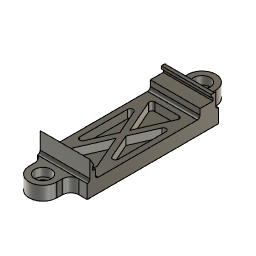
Relay support (Autodesk Fusion 360 design; units mm, degrees)
Autodesk Fusion 360 part; units mm, degrees
sketch "Sketch1" plane through (0, 0, 0) normal (1, 0, 0) x (0, 1, 0)
  line L0 (0, 0) -> (43.2, 0) construction
  line L1 (43.2, 0) -> (43.2, 1.2) construction
  line L2 (43.2, 1.2) -> (0, 1.2) construction
  line L3 (0, 1.2) -> (0, 0) construction
  line L4 (1.3, 0) -> (38.2, 0) construction
  line L5 (38.2, 0) -> (38.2, -2.6) construction
  line L6 (38.2, -2.6) -> (1.3, -2.6) construction
  line L7 (1.3, -2.6) -> (1.3, 0) construction
  line L8 (0.3, 1.4) -> (-1.2, 3.9981)
  line L9 (-1.2, 3.9981) -> (-1.2, -2.1)
  line L10 (-2.2, -3.1) -> (-12.2, -3.1)
  line L11 (-12.2, -3.1) -> (-12.2, -8.1)
  line L12 (-12.2, -8.1) -> (55.4, -8.1)
  line L13 (55.4, -8.1) -> (55.4, -3.1)
  line L14 (55.4, -3.1) -> (45.4, -3.1)
  line L15 (44.4, -2.1) -> (44.4, 1.9)
  line L16 (42.7, 1.4) -> (43.1, 1.4)
  line L17 (43.4, 1.1) -> (43.4, 0)
  line L18 (0.3, 1.4) -> (0.1, 1.4)
  line L19 (-0.2, 1.1) -> (-0.2, 0)
  line L20 (-0.2, 0) -> (0.8, 0)
  line L21 (0.8, 0) -> (0.8, -2.1)
  line L22 (1.8, -3.1) -> (37.7, -3.1)
  line L23 (38.7, -2.1) -> (38.7, 0)
  line L24 (38.7, 0) -> (43.4, 0)
  arc A0 (-2.2, -3.1) -> (-1.2, -2.1) centre (-2.2, -2.1) ccw
  arc A1 (44.4, -2.1) -> (45.4, -3.1) centre (45.4, -2.1) ccw
  arc A2 (0.8, -2.1) -> (1.8, -3.1) centre (1.8, -2.1) ccw
  arc A3 (37.7, -3.1) -> (38.7, -2.1) centre (37.7, -2.1) ccw
  line L25 (42.7, 1.4) -> (42.7, 2.4)
  line L26 (42.7, 2.4) -> (43.9, 2.4)
  arc A4 (43.4, 1.1) -> (43.1, 1.4) centre (43.1, 1.1) ccw
  arc A5 (44.4, 1.9) -> (43.9, 2.4) centre (43.9, 1.9) ccw
  arc A6 (0.1, 1.4) -> (-0.2, 1.1) centre (0.1, 1.1) ccw
  point P0 (43.4, 1.4)
  point P1 (-0.2, 1.4)
  dimension "d1" = 43.2
  dimension "d2" = 1.2
  dimension "d3" = 2.6
  dimension "d4" = 1.3
  dimension "d5" = 5
  dimension "d6" = 5
  dimension "d7" = 0.5
  dimension "d8" = 0.5
  dimension "d9" = 0.5
  dimension "d10" = 0.2
  dimension "d11" = 0.2
  dimension "d12" = 0.2
  dimension "d14" = 1
  dimension "d15" = 1
  dimension "d16" = 60
  dimension "d18" = 0.5
  dimension "d19" = 0.7
  dimension "d20" = 11
  dimension "d21" = 1
  dimension "d22" = 1
  dimension "d25" = 1
  dimension "d26" = 1
  dimension "d59" = 1
  dimension "d60" = 0.3
  dimension "d61" = 0.5
  dimension "d62" = 0.3
  constraint horizontal L0
  constraint vertical L1
  constraint horizontal L2
  constraint vertical L3
  constraint coincident L0.start L3.end
  constraint horizontal L4
  constraint vertical L5
  constraint horizontal L6
  constraint vertical L7
  constraint coincident L0 L4.start
  constraint perpendicular L2 L9
  constraint perpendicular L9 L10
  constraint perpendicular L10 L11
  constraint perpendicular L11 L12
  constraint perpendicular L12 L13
  constraint perpendicular L11 L14
  constraint perpendicular L14 L15
  constraint parallel L14 L16
  constraint perpendicular L14 L17
  constraint parallel L2 L18
  constraint perpendicular L18 L19
  constraint perpendicular L19 L20
  constraint perpendicular L20 L21
  constraint perpendicular L17 L22
  constraint perpendicular L22 L23
  constraint perpendicular L17 L24
  constraint coincident L17 L24.end
  constraint collinear L10 L14
  constraint collinear L0 L24
  constraint collinear L0 L20
  constraint collinear L16 L18
  constraint collinear L10 L22
  constraint tangent L10 A0
  constraint tangent L9 A0
  constraint tangent L15 A1
  constraint tangent L14 A1
  constraint equal L10 L14
  constraint tangent L22 A2
  constraint tangent L21 A2
  constraint tangent L23 A3
  constraint tangent L22 A3
  constraint perpendicular L16 L25
  constraint perpendicular L15 L26
  constraint coincident P0 L16
  constraint coincident P0 L17
  constraint tangent L16 A4
  constraint tangent L17 A4
  constraint tangent L15 A5
  constraint tangent L26 A5
  constraint coincident P1 L18
  constraint coincident P1 L19
  constraint tangent L18 A6
  constraint tangent L19 A6
  measures "d1" distance of L1.end L2.end
  measures "d2" distance of L0.end L1.end
  measures "d3" distance of L4.end L5.end
  measures "d4" distance of L0.start L4.start
  measures "d5" distance of L0.end L4.end
  measures "d6" distance of L12 L22
  measures "d7" distance of L6 L22
  measures "d8" distance of L5 L23
  measures "d9" distance of L7 L21
  measures "d10" distance of L3 L19
  measures "d11" distance of L2 L18
  measures "d12" distance of L1 L17
  measures "d14" distance of L15 L17
  measures "d15" distance of L9 L19
  measures "d16" angle of L8 L18
  measures "d18" distance of L8.start P1
  measures "d19" distance of L16.start P0
  measures "d20" distance of L9 L11
  measures "d21" radius of A0
  measures "d22" radius of A1
  measures "d25" radius of A2
  measures "d26" radius of A3
  measures "d59" distance of L16.start L25.end
  measures "d60" radius of A4
  measures "d61" radius of A5
  measures "d62" radius of A6
extrude "Extrude1" add sketch "Sketch1" along normal blind 18
sketch "Sketch3" plane through (0, 0, -3.1) normal (0, 0, 1) x (-1, 0, 0)
  line L0 (0, -55.4) -> (0, -45.4)
  line L1 (0, -45.4) -> (-18, -45.4)
  line L2 (-18, -45.4) -> (-18, -55.4)
  line L3 (0, -50.4) -> (-18, -50.4) construction
  circle A0 centre (-7, -50.4) radius 1.75
  line L4 (1, -45.4) -> (1, -56.4)
  line L5 (1, -56.4) -> (-19, -56.4)
  line L6 (-19, -56.4) -> (-19, -45.4)
  line L7 (-18, -37.7) -> (-18, -1.8)
  line L8 (-18, 12.2, -5) -> (-18, -55.4, -5)
  line L9 (0, -1.8) -> (0, -37.7)
  arc A1 (-12, -50.4) -> (-2, -50.4) centre (-7, -50.4) ccw
  line L10 (-2, -50.4) -> (-2, -48.4)
  line L11 (-12, -50.4) -> (-12, -48.4)
  arc A2 (0, -45.4) -> (-2, -48.4) centre (1.25, -48.4) ccw
  arc A3 (-12, -48.4) -> (-15, -45.4) centre (-15, -48.4) ccw
  line L12 (0, -45.4) -> (1, -45.4)
  line L13 (-15, -45.4) -> (-19, -45.4)
  line L14 (0, -55.4) -> (-18, -55.4)
  arc A4 through (0, 1.2, 1) (0, 1.4929, 0.2929) (0, 2.2, 0) construction
  line L15 (0, 2.2) -> (-18, 2.2) construction
  arc A5 through (-18, 2.2, 0) (-18, 1.4929, 0.2929) (-18, 1.2, 1) construction
  line L16 (-18, 1.2, 1) -> (0, 1.2, 1) construction
  line L17 (0, -45.4) -> (0, 2.2) construction
  line L18 (0, -21.6) -> (-31.7125, -21.6)
  circle A6 centre (-7, 7.2) radius 1.75
  line L19 (-19, 13.2) -> (-19, 2.2)
  line L20 (-18, 2.2) -> (-18, 12.2)
  arc A7 (-2, 5.2) -> (0, 2.2) centre (1.25, 5.2) ccw
  arc A8 (-2, 7.2) -> (-12, 7.2) centre (-7, 7.2) ccw
  line L21 (0, 12.2) -> (0, 2.2)
  line L22 (-2, 7.2) -> (-2, 5.2)
  line L23 (0, 2.2) -> (-18, 2.2)
  line L24 (0, 7.2) -> (-18, 7.2) construction
  line L25 (-15, 2.2) -> (-19, 2.2)
  line L26 (1, 2.2) -> (1, 13.2)
  line L27 (0, 2.2) -> (1, 2.2)
  line L28 (0, 12.2) -> (-18, 12.2)
  arc A9 (-15, 2.2) -> (-12, 5.2) centre (-15, 5.2) ccw
  line L29 (-12, 7.2) -> (-12, 5.2)
  line L30 (1, 13.2) -> (-19, 13.2)
  dimension "d27" = 7
  dimension "d28" = 3.5
  dimension "d33" = 5
  dimension "d34" = 1
  dimension "d35" = 1
  dimension "d36" = 1
  dimension "d37" = 2
  constraint midpoint L0 L3.start
  constraint midpoint L2 L3.end
  constraint coincident L3 A0.centre
  constraint perpendicular L0 L5
  constraint perpendicular L5 L6
  constraint coincident L3 A1.end
  constraint coincident A0.centre A1.centre
  constraint tangent A1 L10
  constraint tangent A1 L11
  constraint perpendicular L3 L11
  constraint tangent L10 A2
  constraint coincident L0.end L1.start
  constraint tangent L11 A3
  constraint coincident L1 A3.end
  constraint vertical L4
  constraint parallel L1 L13
  constraint collinear L12 L13
  constraint equal L10 L11
  constraint tangent A3 L13
  constraint coincident L15.start L17.end
  constraint midpoint L17 L18.start
  constraint perpendicular L7 L18
  constraint symmetric L0.end L18 L15.start
  constraint symmetric L1.end L18 L15.end
  constraint symmetric L2.end L18 L20.end
  constraint symmetric L3.start L18 L24.start
  constraint symmetric L3.end L18 L24.end
  constraint symmetric A0 L18 A6
  constraint symmetric L4.start L18 L26.start
  constraint symmetric L4.end L18 L26.end
  constraint symmetric L5.end L18 L19.start
  constraint symmetric L0.start L18 L21.start
  constraint symmetric A1.start L18 A8.end
  constraint symmetric A1.end L18 A8.start
  constraint symmetric A1 L18 A8
  constraint symmetric L10.end L18 A7.start
  constraint symmetric L11.end L18 A9.end
  constraint symmetric A2 L18 A7
  constraint symmetric A3.end L18 L25.start
  constraint symmetric A3 L18 A9
  constraint symmetric L6.end L18 L19.end
  measures "d27" distance of L3.start A0.centre
  measures "d28" diameter of A0
  measures "d33" radius of A1
  measures "d34" distance of L5 L14
  measures "d35" distance of L0 L4
  measures "d36" distance of L2 L6
  measures "d37" distance of A1.end L10.end
extrude "Extrude2" cut sketch "Sketch3" against normal blind 6 contours L0 A1 L10 A2 L14 | L1 L2 A1 L11 A3 L13 L14 | A0 | A6 | L20 A8 L23 L25 L28 A9 L29 | A7 A8 L21 L22 L28
sketch "Sketch5" plane through (0, 0, -3.1) normal (0, 0, 1) x (-1, 0, 0)
  line L0 (0, -37.7) -> (0, -1.8)
  line L1 (0, -1.8) -> (-18, -1.8)
  line L2 (-18, -1.8) -> (-18, -37.7)
  line L3 (-18, -37.7) -> (0, -37.7)
  line L4 (-4.623, -35.7) -> (-13.377, -35.7)
  line L5 (-16, -28.4447) -> (-16, -11.0553)
  line L6 (-13.377, -3.8) -> (-4.623, -3.8)
  line L7 (-2, -11.0553) -> (-2, -28.4447)
  line L8 (-2, -3.8) -> (-16, -35.7) construction
  line L9 (-2, -35.7) -> (-16, -3.8) construction
  line L10 (-3.9157, -10.6534) -> (-7.9079, -19.75)
  line L11 (-9, -22.2384) -> (-14.2927, -34.2981)
  line L12 (-3.7073, -34.2981) -> (-9, -22.2384)
  line L13 (-10.0921, -19.75) -> (-14.0843, -10.6534)
  line L14 (-3.9157, -28.8466) -> (-7.9079, -19.75)
  line L15 (-9, -17.2616) -> (-14.2927, -5.2019)
  line L16 (-3.7073, -5.2019) -> (-9, -17.2616)
  line L17 (-10.0921, -19.75) -> (-14.0843, -28.8466)
  arc A0 (-3.7073, -5.2019) -> (-4.623, -3.8) centre (-4.623, -4.8) ccw
  arc A1 (-13.377, -3.8) -> (-14.2927, -5.2019) centre (-13.377, -4.8) ccw
  arc A2 (-14.0843, -10.6534) -> (-16, -11.0553) centre (-15, -11.0553) ccw
  arc A3 (-16, -28.4447) -> (-14.0843, -28.8466) centre (-15, -28.4447) ccw
  arc A4 (-2, -11.0553) -> (-3.9157, -10.6534) centre (-3, -11.0553) ccw
  arc A5 (-3.9157, -28.8466) -> (-2, -28.4447) centre (-3, -28.4447) ccw
  arc A6 (-4.623, -35.7) -> (-3.7073, -34.2981) centre (-4.623, -34.7) ccw
  arc A7 (-14.2927, -34.2981) -> (-13.377, -35.7) centre (-13.377, -34.7) ccw
  line L18 (-2, -3.8) -> (-16, -3.8) construction
  line L19 (-16, -3.8) -> (-16, -35.7) construction
  line L20 (-16, -35.7) -> (-2, -35.7) construction
  line L21 (-2, -35.7) -> (-2, -3.8) construction
  line L22 (0, -19.75) -> (-18, -19.75) construction
  point P0 (-9, -19.75)
  dimension "d40" = 2
  dimension "d41" = 2
  dimension "d42" = 2
  dimension "d43" = 2
  dimension "d48" = 1
  dimension "d49" = 1
  dimension "d50" = 1
  dimension "d51" = 1
  dimension "d52" = 1
  dimension "d53" = 1
  constraint horizontal L4
  constraint vertical L5
  constraint horizontal L6
  constraint vertical L7
  constraint parallel L9 L12
  constraint parallel L9 L14
  constraint parallel L8 L10
  constraint parallel L8 L16
  constraint collinear L10 L11
  constraint collinear L12 L13
  constraint collinear L14 L15
  constraint collinear L16 L17
  constraint tangent L6 A0
  constraint tangent L16 A0
  constraint tangent L6 A1
  constraint tangent L15 A1
  constraint tangent L13 A2
  constraint tangent L5 A2
  constraint equal A1 A2
  constraint tangent L5 A3
  constraint tangent L17 A3
  constraint equal A1 A3
  constraint tangent L10 A4
  constraint tangent L7 A4
  constraint equal A1 A4
  constraint tangent L7 A5
  constraint tangent L14 A5
  constraint equal A1 A5
  constraint tangent L12 A6
  constraint tangent L4 A6
  constraint equal A1 A6
  constraint tangent L4 A7
  constraint tangent L11 A7
  constraint equal A1 A7
  constraint parallel L6 L18
  constraint perpendicular L18 L19
  constraint perpendicular L19 L20
  constraint perpendicular L18 L21
  constraint midpoint L0 L22.start
  constraint midpoint L2 L22.end
  constraint midpoint L22 P0
  constraint coincident L8 P0
  constraint coincident L9 P0
  constraint collinear L4 L20
  constraint collinear L7 L21
  measures "d40" distance of L0 L7
  measures "d41" distance of L2 L5
  measures "d42" distance of L3 L4
  measures "d43" distance of L1 L6
  measures "d48" radius of A0
  measures "d49" radius of A1
  measures "d50" distance of L9 L15
  measures "d51" distance of L9 L13
  measures "d52" distance of L8 L16
  measures "d53" distance of L8 L10
extrude "Extrude3" cut sketch "Sketch5" against normal blind 3 contours L4 L11 L12 A6 A7 | L5 L13 L17 A2 A3 | L6 L15 L16 A0 A1 | L7 L10 L14 A4 A5
sketch "Sketch6" plane through (0, 0, -3.1) normal (0, 0, 1) x (-1, 0, 0)
  arc A0 (-15, 2.2) -> (-12, 5.2) centre (-15, 5.2) ccw
  line L0 (-15, 2.2) -> (0, 2.2)
  arc A1 (-2, 5.2) -> (0, 2.2) centre (1.25, 5.2) ccw
  line L1 (-2, 5.2) -> (-2, 7.2)
  arc A2 (-2, 7.2) -> (-12, 7.2) centre (-7, 7.2) ccw
  line L2 (-12, 7.2) -> (-12, 5.2)
  circle A3 centre (-7, 7.2) radius 1.75
  circle A4 centre (-7, 7.2) radius 3
  circle A5 centre (-7, -50.4) radius 1.75
  circle A6 centre (-7, -50.4) radius 1.75
  circle A7 centre (-7, -50.4) radius 3
  dimension "d56" = 6
  constraint concentric A2 A4
  constraint concentric A6 A7
  constraint equal A4 A7
  measures "d56" diameter of A7
extrude "Extrude4" cut sketch "Sketch6" against normal blind 3 contours A4 | A7
